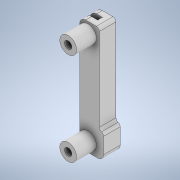
# Autodesk Inventor part: DualPMTController.Spacer.End
Saved by Autodesk Inventor 2022.3 (Build 263350030, 350C)
## iProperties
Created: 2022-08-22
Part Number: DualPMTController.Spacer.End
Material: Generic
Document SubType Name: Modeling
Designer: Graeme
Density: 1 g/cm^3
Appearance: Default
Author: Graeme
Autodesk Inventor part; units mm, degrees
ref_plane "Work Plane1" through (0, 0, 0) normal (0, 0, 1) x (1, 0, 0)
sketch "Sketch1" plane through (0, 0, 0) normal (0, 0, 1) x (1, 0, 0)
  circle A0 centre (43, 15.5) radius 1.55 construction
  circle A1 centre (43, -15.5) radius 1.55 construction
  arc A2 (43, -19) -> (43, -12) centre (43, -15.5) ccw construction
  arc A3 (43, 12) -> (43, 19) centre (43, 15.5) ccw construction
  arc A4 (43, 12) -> (40, 9) centre (43, 9) ccw construction
  line L0 (40, -9) -> (40, 9) construction
  arc A5 (40, -9) -> (43, -12) centre (43, -9) ccw construction
  line L1 (-43, -19) -> (43, -19) construction
  line L2 (43, 19) -> (-43, 19) construction
  line L3 (-43, 19.2) -> (43, 19.2)
  arc A6 (43, 11.8) -> (43, 19.2) centre (43, 15.5) ccw
  arc A7 (43, 11.8) -> (40.2, 9) centre (43, 9) ccw
  line L4 (40.2, 9) -> (40.2, -9)
  arc A8 (40.2, -9) -> (43, -11.8) centre (43, -9) ccw
  arc A9 (43, -19.2) -> (43, -11.8) centre (43, -15.5) ccw
  line L5 (43, -19.2) -> (-43, -19.2)
  line L6 (40.2, 9) -> (40.2, 19.2)
  line L7 (40.2, -9) -> (40.2, -19.2)
  line L8 (40.2, 19.2) -> (48.2, 19.2)
  line L9 (48.2, 19.2) -> (48.2, -19.2)
  line L10 (48.2, -19.2) -> (40.2, -19.2)
  line L11 (40.2, -19.2) -> (40.2, 19.2)
  circle A10 centre (43, 15.5) radius 2.8
  circle A11 centre (43, -15.5) radius 2.8
  point P0 (0, 0)
  dimension "d0" = 0.2
  dimension "d1" = 8
  constraints: 18 end point, 8 point on circle, 6 centre point, 5 point on line, 4 coincident, 2 parallel, 2 tangent, 1 horizontal, 1 perpendicular, 6 other
  measures "d0" distance between parallel lines of L0 L4
  measures "d1" distance of L9.end L10.end
ref_plane "Work Plane2" through (-378.6125, -20.325, 8.6441) normal (0, 0, -1) x (0, 1, 0)
extrude "Extrusion1" add sketch "Sketch1" along normal up to surface (8.6441 mm away) contours A10 | A11
ref_plane "Work Plane3" through (-380.1125, -20.825, 444.0892) normal (0, 1, 0) x (-1, 0, 0)
ref_plane "Work Plane4" through (0, 0, 0) normal (0, 0, 1) x (1, 0, 0)
sketch "Sketch2" plane through (0, 0, 0) normal (0, 0, 1) x (1, 0, 0)
  arc A0 (43, 12) -> (43, 19) centre (43, 15.5) ccw projected
  arc A1 (43, -19) -> (43, -12) centre (43, -15.5) ccw projected
  line L0 (40.2, 19) -> (48.2, 19)
  line L1 (48.2, 19) -> (48.2, -19)
  line L2 (48.2, -19) -> (40.2, -19)
  line L3 (40.2, -19) -> (40.2, 19)
  circle A2 centre (43, 15.5) radius 2.8 projected
  point P0 (0, 0)
  point P1 (40.2, 15.5)
  dimension "d4" = 8
  constraints: 8 end point, 3 tangent, 2 parallel, 1 horizontal, 1 perpendicular
  measures "d4" distance of L1.end L2.end
extrude "Extrusion2" add sketch "Sketch2" along normal blind 2
ref_plane "Work Plane5" through (0, 0, -1.5518) normal (0, 0, -1) x (-1, 0, 0)
sketch "Sketch3" plane through (0, 0, -1.5518) normal (0, 0, -1) x (-1, 0, 0)
  arc A0 (-43, 19) -> (-43, 12) centre (-43, 15.5) ccw projected
  arc A1 (-40, 9) -> (-43, 12) centre (-43, 9) ccw projected
  line L0 (-40, -9) -> (-40, 9) projected
  arc A2 (-43, -12) -> (-40, -9) centre (-43, -9) ccw projected
  arc A3 (-43, -12) -> (-43, -19) centre (-43, -15.5) ccw projected
  arc A4 (-43, 19.2) -> (-43, 11.8) centre (-43, 15.5) ccw
  arc A5 (-40.2, 9) -> (-43, 11.8) centre (-43, 9) ccw
  line L1 (-40.2, 9) -> (-40.2, -9)
  arc A6 (-43, -11.8) -> (-40.2, -9) centre (-43, -9) ccw
  arc A7 (-43, -11.8) -> (-43, -19.2) centre (-43, -15.5) ccw
  line L2 (-48.2, -19) -> (-48.2, 19) projected
  line L3 (-48.2, 19) -> (-44.2, 19)
  line L4 (-48.2, 19) -> (-40.2, 19) projected
  line L5 (-40.2, -19) -> (-48.2, -19) projected
  line L6 (-48.2, 19) -> (-48.2, -19)
  line L7 (-48.2, -19) -> (-44.2, -19)
  point P0 (0, 0)
  point P1 (-44.2, -19)
  dimension "d7" = 0.2
  constraints: 8 end point, 8 point on circle, 4 centre point, 2 midpoint, 1 vertical, 4 other
  measures "d7" radial gap between concentric circles of A0 A4
extrude "Extrusion3" add sketch "Sketch3" against normal up to surface (1.5518 mm away) contours A4 A5 L1 A6 A7 L5 L2 L3
sketch "Sketch4" plane through (0, 0, -1.5518) normal (0, 0, -1) x (-1, 0, 0)
  line L0 (-48.2, -19) -> (-48.2, 19) projected
  line L1 (-40.2, -9) -> (-40.2, -19) projected
  line L2 (-48.2, 19) -> (-40.2, 19)
  line L3 (-40.2, 19) -> (-40.2, -19)
  line L4 (-40.2, -19) -> (-48.2, -19)
  line L5 (-48.2, -19) -> (-48.2, 19)
  point P0 (0, 0)
  constraints: 8 end point, 2 parallel, 1 horizontal, 1 perpendicular
extrude "Extrusion4" add sketch "Sketch4" along normal blind 2
fillet "Fillet1" radius 2 6 edges at (40.2, 19, -2.5518) (40.2, 19, 1) (48.2, 19, -0.7759) (40.2, -19, -2.5518) (40.2, -19, 1) (48.2, -19, -0.7759)
sketch "Sketch5" plane through (43, 15.5, 8.6441) normal (0, 0, 1) x (1, 0, 0)
  circle A0 centre (0, 0) radius 2.8 projected
  circle A1 centre (0, -31) radius 2.8 projected
  circle A2 centre (0, -31) radius 2.8 projected
  point P0 (-43, -15.5)
  point P1 (-2.8, -31)
  constraints: 2 coincident, 2 horizontal alignment
hole "Hole1" at (43, 15.5, 8.6441) at (43, -15.5, 8.6441) direction (0, 0, -1) diameter 2.459 end through all thread size "M3x0.5" class "6H" standard "ISO Metric profile"
sketch "Sketch6" plane through (0, 0, 2) normal (0, 0, 1) x (1, 0, 0)
  ellipse E0 centre (47.6779, 18.325) end of major axis (47.6779, 20.325) minor radius 0.684 (47.4573, 20.2182) -> (46.9938, 18.325) ccw projected
  line L0 (46.9938, 18.325) -> (46.9938, 15.1412) projected
  ellipse E1 centre (47.6779, 15.1412) end of major axis (47.6779, 13.1412) minor radius 0.684 (46.9938, 15.1412) -> (47.4439, 13.2618) ccw projected
  line L1 (47.4875, 13.1421) -> (47.4875, 11.797) projected
  line L2 (48.4875, 10.428) -> (47.4875, 10.428) projected
  line L3 (47.4875, 10.428) -> (47.4875, -10.428) projected
  spline S0 degree 3 poles (47.4875, -10.428) (47.4875, -10.4446) (47.514, -10.4613) (47.6162, -10.4947) (47.6918, -10.5113) (47.8806, -10.5447) (47.9938, -10.5614) (48.2405, -10.5947) (48.374, -10.6114) (48.5075, -10.6281) knots 0 0 0 0 0.25 0.25 0.5 0.5 0.75 0.75 1 1 1 1 projected
  spline S1 degree 3 poles (48.5075, 11.5969) (48.374, 11.6136) (48.2405, 11.6303) (47.9938, 11.6636) (47.8806, 11.6803) (47.6918, 11.7137) (47.6162, 11.7303) (47.514, 11.7637) (47.4875, 11.7804) (47.4875, 11.797) knots 0 0 0 0 0.25 0.25 0.5 0.5 0.75 0.75 1 1 1 1 projected
  line L4 (48.2, -17) -> (48.2, 17) projected
  line L5 (48.2, -10.789) -> (46.7938, -10.789)
  line L6 (46.7938, -10.789) -> (46.7938, 18.9098)
  line L7 (46.7938, 18.9098) -> (48.2, 18.9098)
  line L8 (48.2, 18.9098) -> (48.2, -10.789)
  arc A0 (48.2, 17) -> (46.2, 19) centre (46.2, 17) ccw projected
  point P0 (0, 0)
  point P1 (48.2, -10.589)
  dimension "d20" = 0.2
  dimension "d21" = 0.2
  constraints: 8 end point, 2 parallel, 2 point on line, 1 horizontal, 1 perpendicular, 1 point on circle, 3 other
  measures "d20" distance between parallel lines of L6 L0
  measures "d21" distance from line of L5 point (48.2, -10.589)
extrude "Extrusion5" cut sketch "Sketch6" against normal through all contours A0 L4 L2 L3 S0 L5 L6 | L4 S0 L3 L2
fillet "Fillet2" radius 1 3 edges at (48.2, -10.789, -0.7759) (46.7938, -10.789, -0.7759) (46.7938, 18.9098, -0.7759)
